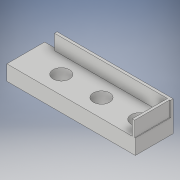
# Autodesk Inventor part: Part3
Saved by Autodesk Inventor 2019 (Build 230136000, 136)
## iProperties
Created: 2020-02-19
Part Number: Part3
Material: Generic
Document SubType Name: Modeling
Designer: Lenovo
Density: 1 g/cm^3
Appearance: Default
Author: Lenovo
Autodesk Inventor part; units mm, degrees
ref_plane "YZ Plane" through (0, 0, 0) normal (1, 0, 0) x (0, 1, 0)
ref_plane "XZ Plane" through (0, 0, 0) normal (0, 1, 0) x (-1, 0, 0)
ref_plane "XY Plane" through (0, 0, 0) normal (0, 0, 1) x (1, 0, 0)
sketch "Sketch1" plane through (0, 0, 0) normal (0, 1, 0) x (-1, 0, 0)
  line L0 (0, 0) -> (-340, 0)
  line L1 (-340, 0) -> (-340, -100)
  line L2 (-340, -100) -> (0, -100)
  line L3 (0, -100) -> (0, 0)
  dimension "d0" = 340
  dimension "d1" = 100
  constraints: 8 end point, 2 parallel, 1 horizontal, 1 perpendicular
  measures "d0" distance of L2.end L1.end
  measures "d1" distance of L1.end L0.end
extrude "Extrusion1" add sketch "Sketch1" along normal blind 40
sketch "Sketch2" plane through (0, 40, 0) normal (0, 1, 0) x (1, 0, 0)
  circle A0 centre (302.5068, 47.875) radius 21.6916
  circle A1 centre (202.5481, 47.875) radius 21.6916
  circle A2 centre (96.2761, 47.875) radius 21.6916
  circle A3 centre (302.5068, 47.875) radius 21.6916
  point P0 (0, 0)
  constraints: 4 centre point
extrude "Extrusion2" cut sketch "Sketch2" against normal blind 500
sketch "Sketch3" plane through (0, 40, 0) normal (0, 1, 0) x (1, 0, 0)
  line L0 (340, 100) -> (0, 100) projected
  line L1 (33.1442, 93.1195) -> (340, 93.1195)
  line L2 (340, 93.1195) -> (340, 100)
  line L3 (340, 100) -> (33.1442, 100)
  line L4 (33.1442, 100) -> (33.1442, 93.1195)
  point P0 (0, 0)
  constraints: 8 end point, 2 parallel, 1 horizontal, 1 perpendicular
extrude "Extrusion3" add sketch "Sketch3" along normal blind 40
sketch "Sketch4" plane through (0, 40, 0) normal (0, 1, 0) x (1, 0, 0)
  line L0 (340, 93.1195) -> (33.1442, 93.1195) projected
  line L1 (338.2816, 0) -> (331.9684, 0)
  line L2 (331.9684, 0) -> (331.9684, 93.1195)
  line L3 (331.9684, 93.1195) -> (338.2816, 93.1195)
  line L4 (338.2816, 93.1195) -> (338.2816, 0)
  point P0 (0, 0)
  constraints: 8 end point, 2 parallel, 1 horizontal, 1 perpendicular, 1 point on line
extrude "Extrusion4" add sketch "Sketch4" along normal blind 40
body "Solid1"
